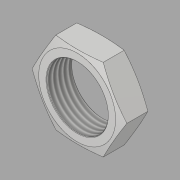
# Autodesk Inventor part: AN924-8D
Saved by Autodesk Inventor 2019 (Build 230136000, 136)
## iProperties
Created: 2018-11-23
Part Number: AN924-8D
Material: Aluminum 2014-T6
Document SubType Name: Modeling
Designer: erics
Mass: 5.92106 g
Surface Area: 16.5239 cm^2
Volume: 2.1228 cm^3
Density: 2.78927 g/cm^3
Appearance: Satin
Author: erics
Autodesk Inventor part; units mm, degrees
ref_plane "YZ Plane" through (0, 0, 0) normal (1, 0, 0) x (0, 1, 0)
ref_plane "XZ Plane" through (0, 0, 0) normal (0, 1, 0) x (-1, 0, 0)
ref_plane "XY Plane" through (0, 0, 0) normal (0, 0, 1) x (1, 0, 0)
sketch "Sketch1" plane through (0, 0, 0) normal (0, 0, 1) x (1, 0, 0)
  line L0 (-7.3323, 12.7) -> (7.3323, 12.7)
  line L1 (7.3323, 12.7) -> (14.6647, 0)
  line L2 (14.6647, 0) -> (7.3323, -12.7)
  line L3 (7.3323, -12.7) -> (-7.3323, -12.7)
  line L4 (-7.3323, -12.7) -> (-14.6647, 0)
  line L5 (-14.6647, 0) -> (-7.3323, 12.7)
  circle A0 centre (0, 0) radius 9.525
  dimension "d0" = 25.4
  dimension "d1" = 19.05
  constraints: 12 end point, 2 coincident, 1 centre point, 1 horizontal, 13 other
  measures "d0" distance between parallel lines of L0 L3
  measures "d1" diameter of A0
extrude "Extrusion1" add sketch "Sketch1" along normal mid plane 7.9502
chamfer "Chamfer1" distance 0.127 angle 45 2 edges at (-9.525, 0, 3.9751) (-9.525, 0, -3.9751)
sketch "Sketch2" plane through (0, 0, 0) normal (0, 1, 0) x (-1, 0, 0)
  line L0 (11.8999, 3.9751) -> (14.6647, 3.2343)
  line L1 (14.6647, 3.2343) -> (14.6647, 3.9751)
  line L2 (14.6647, 3.9751) -> (11.8999, 3.9751)
  line L3 (14.6647, 3.9751) -> (7.3323, 3.9751) construction
  line L4 (7.3323, 3.9751) -> (7.3323, -3.9751) construction
  line L5 (14.6647, 3.9751) -> (7.3323, 3.9751) construction
  line L6 (14.6647, 3.9751) -> (14.6647, -3.9751) construction
  line L7 (7.3323, -3.9751) -> (14.6647, -3.9751) construction
  line L8 (0, 0) -> (14.6647, 0) construction
  line L9 (11.8999, -3.9751) -> (14.6647, -3.2343)
  line L10 (14.6647, -3.2343) -> (14.6647, -3.9751)
  line L11 (14.6647, -3.9751) -> (11.8999, -3.9751)
  line L12 (0, -3.8938) -> (0, 3.8938) projected
  dimension "d7" = 11.8999
  dimension "d8" = 15
  constraints: 14 end point, 5 symmetric about line, 2 point on line, 1 midpoint, 1 perpendicular, 1 vertical
  measures "d7" horizontal distance of L0.start L8.start
  measures "d8" angle of L2 L0
revolve "Revolution1" cut sketch "Sketch2" angle 360 about axis through (0, 0, -10) along (0, 0, 1)
thread "Thread1" size "3/4-16 UNF" class "3B" standard "ANSI Unified Screw Threads" full length
equation "\"d0\" = AN924_A"
equation "\"d1\" = AN924_T"
equation "\"d2\" = AN924_B"
equation "\"d7\" = 0.5 * AN924_G"
equation "\"AN924_A\" = 25.4"
equation "\"AN924_B\" = 7.9502"
equation "\"AN924_G\" = 23.7998"
equation "\"AN924_T\" = 19.05"
equation "\"Tube_OD\" = 12.7"
body "Solid1"
